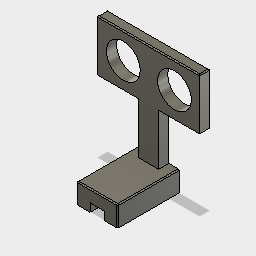
FinalUltrasonic v4 (Autodesk Fusion 360 design; units mm, degrees)
Autodesk Fusion 360 part; units mm, degrees
sketch "Sketch1" plane through (0, 0, 0) normal (0, 0, 1) x (1, 0, 0)
  line L0 (-20, 75) -> (30, 75)
  line L1 (30, 75) -> (30, 50)
  line L2 (30, 50) -> (-20, 50)
  line L3 (-20, 50) -> (-20, 75)
  line L4 (0, 50) -> (10, 50)
  line L5 (10, 50) -> (10, 25)
  line L6 (10, 25) -> (0, 25)
  line L7 (0, 25) -> (0, 50)
  line L8 (-5, 25) -> (15, 25)
  line L9 (15, 25) -> (15, 15)
  line L10 (15, 15) -> (-5, 15)
  line L11 (-5, 15) -> (-5, 25)
  dimension "d1" = 50
  dimension "d2" = 25
  measures "d1" distance of L0.start L0.end
  measures "d2" distance of L0.start L2.end
extrude "Extrude1" add sketch "Sketch1" along normal blind 5
move_body "Move1" bodies 1 to x (1, 0, 0) y (0, 1, 0) z (0, 0, 1) at (-5.1821, -16.3235, 0)
move_body "Move2" bodies 1 to x (1, 0, 0) y (0, 1, 0) z (0, 0, 1) at (-0.5182, 0, -1.0364)
sketch "Sketch2" plane through (0, 0, 3.9636) normal (0, 0, 1) x (1, 0, 0)
  line L0 (-10.7003, -1.3235) -> (9.2997, -1.3235)
  line L1 (9.2997, -1.3235) -> (9.2997, 8.6765)
  line L2 (9.2997, 8.6765) -> (4.2997, 8.6765)
  line L3 (4.2997, 8.6765) -> (4.2997, 33.6765)
  line L4 (4.2997, 33.6765) -> (24.2997, 33.6765)
  line L5 (24.2997, 33.6765) -> (24.2997, 58.6765)
  line L6 (24.2997, 58.6765) -> (-25.7003, 58.6765)
  line L7 (-25.7003, 58.6765) -> (-25.7003, 33.6765)
  line L8 (-25.7003, 33.6765) -> (-5.7003, 33.6765)
  line L9 (-5.7003, 33.6765) -> (-5.7003, 8.6765)
  line L10 (-5.7003, 8.6765) -> (-10.7003, 8.6765)
  line L11 (-10.7003, 8.6765) -> (-10.7003, -1.3235)
  circle A0 centre (-13, 46) radius 8.25
  circle A1 centre (12, 46) radius 8.25
  line L12 (2.7978, 2.6677) -> (-4.2022, 2.6677)
  line L13 (-4.2022, 2.6677) -> (-4.2022, -1.3323)
  line L14 (-4.2022, -1.3323) -> (2.7978, -1.3323)
  line L15 (2.7978, -1.3323) -> (2.7978, 2.6677)
  line L16 (-10.7003, 8.6765) -> (-4.2022, 8.6765)
  line L17 (-4.2022, 8.6765) -> (-4.2022, -1.3323)
  line L18 (-4.2022, -1.3323) -> (-10.7003, -1.3323)
  line L19 (-10.7003, -1.3323) -> (-10.7003, 8.6765)
  line L20 (-4.2022, 8.6765) -> (2.7978, 8.6765)
  line L21 (2.7978, 8.6765) -> (2.7978, 2.6677)
  line L22 (2.7978, 2.6677) -> (-4.2022, 2.6677)
  line L23 (-4.2022, 2.6677) -> (-4.2022, 8.6765)
  line L24 (2.7978, 8.6765) -> (9.2997, 8.6765)
  line L25 (9.2997, 8.6765) -> (9.2997, -1.3235)
  line L26 (9.2997, -1.3235) -> (2.7978, -1.3235)
  line L27 (2.7978, -1.3235) -> (2.7978, 8.6765)
  dimension "d5" = 16.5
  dimension "d6" = 16.5
  dimension "d11" = 7
  dimension "d12" = 4
  measures "d5" diameter of A0
  measures "d6" diameter of A1
  measures "d11" distance of L12.start L12.end
  measures "d12" distance of L12.start L14.end
extrude "Extrude5" add sketch "Sketch2" along normal blind 25 contours L0 L1 L2 L15 L21 L24 L25 L26 L27 | L0 L10 L11 L13 L16 L17 L19 L23 | L12 L17 L20 L21 L22 L23 L27
extrude "Extrude4" cut sketch "Sketch2" against normal blind 17 contours L0 L12 L13 L15 L17 L22 L27
extrude "Extrude2" cut sketch "Sketch2" against normal blind 7 contours A0
extrude "Extrude3" cut sketch "Sketch2" against normal blind 9 contours A1
fillet "Fillet1" radius 0.5 6 edges at (9.2997, 8.6765, 13.9636) (-10.7003, 8.6765, 13.9636) (-0.7003, 58.6765, 3.9636) (-0.7003, 58.6765, -1.0364) (24.2997, 58.6765, 1.4636) (-25.7003, 58.6765, 1.4636)
fillet "Fillet2" radius 0.5 5 edges at (9.2997, 3.4265, 28.9636) (9.1533, 8.53, 28.9636) (-0.7003, 8.6765, 28.9636) (-10.5538, 8.53, 28.9636) (-10.7003, 3.4265, 28.9636)
